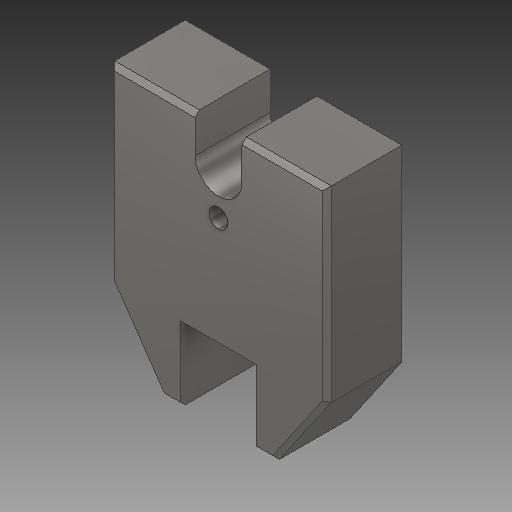
# Autodesk Inventor part: Base
Saved by Autodesk Inventor 2018 (Build 220112000, 112)
## iProperties
Created: 2017-12-20
Part Number: Base
Material: Stainless Steel
Document SubType Name: Modeling
Designer: 232963
Density: 8 g/cm^3
Appearance: Semi-Polished
Mass: 1026.23 g
Surface Area: 205.529 cm^2
Volume: 128.279 cm^3
Author: 232963
Autodesk Inventor part; units mm, degrees
ref_plane "YZ Plane" through (0, 0, 0) normal (1, 0, 0) x (0, 1, 0)
ref_plane "XZ Plane" through (0, 0, 0) normal (0, 1, 0) x (-1, 0, 0)
ref_plane "XY Plane" through (0, 0, 0) normal (0, 0, 1) x (1, 0, 0)
sketch "Sketch1" plane through (0, 0, 0) normal (0, 0, 1) x (1, 0, 0)
  line L0 (73.279, 0) -> (73.279, 88.9)
  line L1 (0, 88.9) -> (0, 0)
  arc A0 (28.702, 76.2) -> (44.577, 76.2) centre (36.6395, 76.2) ccw
  line L2 (28.702, 76.2) -> (28.702, 88.9)
  line L3 (44.577, 76.2) -> (44.577, 88.9)
  line L4 (73.279, 88.9) -> (44.577, 88.9)
  line L5 (28.702, 88.9) -> (0, 88.9)
  line L6 (23.8252, 0) -> (49.4538, 0)
  line L7 (49.4538, 0) -> (49.4538, 25.4)
  line L8 (49.4538, 25.4) -> (23.8252, 25.4)
  line L9 (23.8252, 25.4) -> (23.8252, 0)
  line L10 (0, 25.4) -> (17.526, 0)
  line L11 (73.279, 25.4) -> (55.753, 0)
  line L12 (0, 0) -> (23.8252, 0)
  line L13 (49.4538, 0) -> (73.279, 0)
  dimension "d0" = 73.279
  dimension "d1" = 88.9
  dimension "d2" = 15.875
  dimension "d4" = 25.6286
  dimension "d5" = 63.5
  dimension "d6" = 23.8252
  dimension "d7" = 17.526
  dimension "d8" = 17.526
  constraints: 28 end point, 7 parallel, 7 perpendicular, 4 point on line, 3 horizontal, 2 point on circle, 2 tangent, 1 centre point
  measures "d0" distance of L1.start L0.end
  measures "d1" distance of L0.end L0.start
  measures "d2" diameter of A0
  measures "d4" distance of L8.end L7.end
  measures "d5" distance between parallel lines of L5 L8
  measures "d6" distance between parallel lines of L1 L9
  measures "d7" distance of L1.end L10.end
  measures "d8" distance of L0.start L11.end
extrude "Extrusion1" add sketch "Sketch1" along normal blind 25.4 contours L11 L13 L7 L8 L9 L12 L10 L1 L5 L2 A0 L3 L4 L0
sketch "Sketch2" plane through (0, 0, 25.4) normal (0, 0, 1) x (1, 0, 0)
  circle A0 centre (36.6395, 61.9252) radius 3.2385
  line L0 (73.279, 25.4) -> (73.279, 88.9) projected
  line L1 (0, 88.9) -> (0, 25.4) projected
  line L2 (73.279, 88.9) -> (44.577, 88.9) projected
  point P0 (0, 0)
  dimension "d12" = 73.279
  dimension "d13" = 36.6395
  dimension "d14" = 6.477
  dimension "d15" = 26.9748
  constraints: 1 centre point
  measures "d12" distance between parallel lines of L0 L1
  measures "d13" distance from line of L0 A0.centre
  measures "d14" diameter of A0
  measures "d15" distance from line of L2 A0.centre
extrude "Extrusion2" cut sketch "Sketch2" against normal blind 14.2748
sketch "Sketch3" plane through (23.8252, 25.4, 0) normal (0, -1, 0) x (1, 0, 0)
  line L0 (0, 25.4) -> (25.6286, 25.4) projected
  line L1 (25.6286, 0) -> (25.6286, 25.4) projected
  point P0 (-23.8252, 0)
  point P1 (12.8143, 12.7)
  dimension "d18" = 12.7
  dimension "d19" = 12.8143
  dimension "d20" = 25.6286
  measures "d18" distance from line of L0 point (12.814, 12.7)
  measures "d19" distance from line of L1 point (12.814, 12.7)
  measures "d20" distance of L0.start L0.end
hole "Hole1" at (36.6395, 25.4, 12.7) direction (0, 1, 0) diameter 7.7978 depth 19.05 tip angle 118 thread size "3/8-16 UNC" class "2B" standard "ANSI Unified Screw Threads"
chamfer "Chamfer1" distance 1.524 angle 45 8 edges at (14.351, 88.9, 25.4) (0, 57.15, 25.4) (8.763, 12.7, 25.4) (20.6756, 0, 25.4) (52.6034, 0, 25.4) (64.516, 12.7, 25.4) (73.279, 57.15, 25.4) (58.928, 88.9, 25.4)
equation "\"d13\" = 0.5 * d12"
equation "\"d19\" = 0.5 * d20"
body "Solid1"
